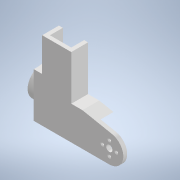
# Autodesk Inventor part: bodyR
Saved by Autodesk Inventor 2020 (Build 240168000, 168)
## iProperties
Created: 2020-01-03
Part Number: bodyR
Material: Generic
Document SubType Name: Modeling
Designer: my
Density: 1 g/cm^3
Appearance: Default
Author: my
Autodesk Inventor part; units mm, degrees
ref_plane "YZ Plane" through (0, 0, 0) normal (1, 0, 0) x (0, 1, 0)
ref_plane "XZ Plane" through (0, 0, 0) normal (0, 1, 0) x (-1, 0, 0)
ref_plane "XY Plane" through (0, 0, 0) normal (0, 0, 1) x (1, 0, 0)
sketch "Sketch1" plane through (0, 0, 0) normal (0, 0, 1) x (1, 0, 0)
  line L0 (0, 0) -> (120, 0)
  line L1 (52, 60) -> (52, 140)
  line L2 (0, 80) -> (0, 140)
  circle A0 centre (120, 29) radius 29
  line L3 (52, 60) -> (72, 60)
  line L4 (72, 60) -> (121.1925, 57.9755)
  line L5 (0, 140) -> (52, 140)
  line L6 (0, 80) -> (-15, 80)
  line L7 (-15, 80) -> (-15, 0)
  line L8 (-15, 0) -> (0, 0)
  dimension "d4" = 52
  dimension "d6" = 58
  dimension "d7" = 20
  dimension "d8" = 80
  dimension "d12" = 120
  dimension "d14" = 15
  dimension "d15" = 80
  dimension "d17" = 60
  constraints: 18 end point, 4 horizontal, 2 parallel, 2 point on circle, 2 tangent, 2 vertical, 1 centre point, 1 coincident, 1 horizontal alignment, 1 perpendicular
  measures "d4" distance between parallel lines of L1 L2
  measures "d6" diameter of A0
  measures "d7" distance of L1.start L3.end
  measures "d8" distance of L1.start L1.end
  measures "d12" distance of L0.start L0.end
  measures "d14" distance of L7.end L0.start
  measures "d15" distance of L6.end L7.end
  measures "d17" distance between parallel lines of L0 L3
extrude "Extrusion1" add sketch "Sketch1" along normal blind 30
shell "Shell1" thickness 7 removed faces 2 at (34.6667, 140, 10) at (57.3333, 20, 0)
sketch "Sketch3" plane through (-15, 0, 0) normal (-1, 0, 0) x (0, 0, 1)
  line L0 (0, 80) -> (0, 0) projected
  circle A0 centre (0, 40) radius 26
  line L1 (0, 0) -> (30, 0) projected
  dimension "d16" = 52
  constraints: 1 centre point, 1 midpoint
  measures "d16" diameter of A0
extrude "Extrusion2" add sketch "Sketch3" along normal mid plane 30
sketch "Sketch4" plane through (0, 0, 0) normal (1, 0, 0) x (0, 0, -1)
  arc A0 (-23, 27.8756) -> (-23, 52.1244) centre (0, 40) ccw projected
  circle A1 centre (0, 40) radius 20
  point P0 (0, 0)
  dimension "d22" = 40
  constraints: 1 centre point, 1 coincident
  measures "d22" diameter of A1
extrude "Extrusion3" cut sketch "Sketch4" against normal blind 20
sketch "Sketch5" plane through (-20, 40, 0) normal (1, 0, 0) x (0, 0, -1)
  circle A0 centre (0, 0) radius 12.5
  circle A1 centre (0, 0) radius 20 projected
  point P0 (0, -40)
  point P1 (0, 12.5)
  point P2 (-12.5, 0)
  point P3 (0, -12.5)
  point P4 (12.5, 0)
  dimension "d25" = 25
  constraints: 4 point on circle, 1 centre point, 1 concentric
  measures "d25" diameter of A0
hole "Hole1" at (-20, 52.5, 0) at (-20, 40, 12.5) at (-20, 27.5, 0) at (-20, 40, -12.5) direction (-1, 0, 0) diameter 3.4 depth 20 countersink diameter 6.3 countersink angle 90 clearance for "Countersunk Flat Head Screw ISO 2009/7046" size "M3" standard "ISO"
sketch "Sketch6" plane through (-20, 40, 0) normal (1, 0, 0) x (0, 0, -1)
  circle A0 centre (4, -4) radius 2
  circle A1 centre (9.5, -9.5) radius 3.25
  line L0 (0, 0) -> (9.5, -9.5) construction
  line L1 (0, 0) -> (4, 0) construction
  line L2 (4, 0) -> (4, -4) construction
  line L3 (4, -4) -> (0, -4)
  line L4 (0, -4) -> (0, 0) construction
  circle A2 centre (0, 0) radius 20 projected
  circle A3 centre (0, 0) radius 4 construction
  circle A4 centre (4, 4) radius 2
  circle A5 centre (9.5, 9.5) radius 3.25
  circle A6 centre (-4, 4) radius 2
  circle A7 centre (-9.5, 9.5) radius 3.25
  circle A8 centre (-4, -4) radius 2
  circle A9 centre (-9.5, -9.5) radius 3.25
  point P0 (0, -40)
  dimension "d39" = 8
  dimension "d33" = 4
  dimension "d34" = 6.5
  dimension "d36" = 4
  dimension "d37" = 4
  dimension "d38" = 5.5
  dimension "d42" = 360
  constraints: 10 end point, 8 centre point, 3 coincident, 2 parallel, 1 horizontal, 1 horizontal alignment, 1 perpendicular, 1 point on line, 1 vertical, 21 other
  measures "d33" diameter of A0
  measures "d34" diameter of A1
  measures "d36" distance of L1.end L2.end
  measures "d37" distance of L2.end L3.end
  measures "d38" horizontal distance of L0.end L2.end
extrude "Extrusion4" cut sketch "Sketch6" against normal blind 10 contours A0 | A1 | A4 | A5 | A6 | A7 | A8 | A9
sketch "Sketch7" plane through (120, 7, 23) normal (0, 0, -1) x (-1, 0, 0)
  arc A0 (-0.9046, 43.9814) -> (0, 0) centre (0, 22) ccw projected
  circle A1 centre (0, 22) radius 40.5
  point P0 (120, -7)
  dimension "d46" = 81
  constraints: 1 centre point, 1 coincident
  measures "d46" diameter of A1
extrude "Extrusion5" cut sketch "Sketch7" along normal through all
sketch "Sketch8" plane through (0, 0, 30) normal (0, 0, 1) x (1, 0, 0)
  arc A0 (120, 0) -> (121.1925, 57.9755) centre (120, 29) ccw projected
  circle A1 centre (120, 29) radius 12.5
  point P0 (0, 0)
  point P1 (120, 16.5)
  point P2 (107.5, 28.9999)
  point P3 (120, 41.5)
  point P4 (132.5, 28.9999)
  dimension "d49" = 25
  constraints: 4 point on circle, 1 centre point, 1 coincident
  measures "d49" diameter of A1
hole "Hole2" at (120, 16.5, 30) at (107.5, 28.9999, 30) at (120, 41.5, 30) at (132.5, 28.9999, 30) direction (0, 0, -1) diameter 3.4 depth 20 countersink diameter 6.3 countersink angle 90 clearance for "Countersunk Flat Head Screw ISO 2009/7046" size "M3" standard "ISO"
sketch "Sketch9" plane through (0, 0, 30) normal (0, 0, 1) x (1, 0, 0)
  arc A0 (120, 0) -> (121.1925, 57.9755) centre (120, 29) ccw projected
  circle A1 centre (120, 29) radius 5.5
  point P0 (0, 0)
  dimension "d57" = 11
  constraints: 1 centre point, 1 coincident
  measures "d57" diameter of A1
extrude "Extrusion6" cut sketch "Sketch9" against normal through all
body "Solid1"
